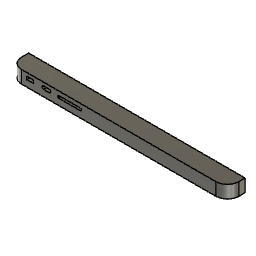
laptop side reference model v4 (Autodesk Fusion 360 design; units mm, degrees)
Autodesk Fusion 360 part; units mm, degrees
sketch "Sketch1" plane through (0, 0, 0) normal (0, 0, 1) x (1, 0, 0) in component "Laptop side"
  line L0 (0, 0) -> (225.9, 0)
  line L1 (225.9, 0) -> (225.9, 18.5)
  line L2 (225.9, 18.5) -> (0, 18.5)
  line L3 (0, 18.5) -> (0, 0)
  dimension "d1" = 225.9
  dimension "d2" = 18.5
  constraint horizontal L0
  constraint vertical L1
  constraint horizontal L2
  constraint vertical L3
  constraint coincident L0.start L3.end
  measures "d1" distance of L0.start L0.end
  measures "d2" distance of L0.end L1.end
extrude "Extrude1" add sketch "Sketch1" along normal blind 13.24 in component "Laptop side"
sketch "Sketch2" plane through (0, 0, 0) normal (0, -1, 0) x (1, 0, 0) in component "Laptop side"
  line L0 (0, 0) -> (225.9, 0)
  line L1 (225.9, 0) -> (225.9, 13.24)
  line L2 (225.9, 13.24) -> (0, 13.24)
  line L3 (0, 13.24) -> (0, 0)
  line L4 (16.56, 9.86) -> (23.66, 9.86)
  line L5 (23.66, 9.86) -> (23.66, 6.76)
  line L6 (23.66, 6.76) -> (16.56, 6.76)
  line L7 (16.56, 6.76) -> (16.56, 9.86)
  line L8 (33.96, 9.82) -> (40.16, 9.82)
  line L9 (41.56, 8.42) -> (41.56, 8.04)
  line L10 (40.16, 6.64) -> (33.96, 6.64)
  line L11 (32.56, 8.04) -> (32.56, 8.42)
  arc A0 (33.96, 9.82) -> (32.56, 8.42) centre (33.96, 8.42) ccw
  arc A1 (32.56, 8.04) -> (33.96, 6.64) centre (33.96, 8.04) ccw
  arc A2 (40.16, 6.64) -> (41.56, 8.04) centre (40.16, 8.04) ccw
  arc A3 (41.56, 8.42) -> (40.16, 9.82) centre (40.16, 8.42) ccw
  line L12 (49.66, 9.04) -> (72.76, 9.04)
  line L13 (73.46, 8.34) -> (73.46, 7.34)
  line L14 (72.76, 6.64) -> (49.66, 6.64)
  line L15 (48.96, 7.34) -> (48.96, 8.34)
  arc A4 (49.66, 9.04) -> (48.96, 8.34) centre (49.66, 8.34) ccw
  arc A5 (48.96, 7.34) -> (49.66, 6.64) centre (49.66, 7.34) ccw
  arc A6 (72.76, 6.64) -> (73.46, 7.34) centre (72.76, 7.34) ccw
  arc A7 (73.46, 8.34) -> (72.76, 9.04) centre (72.76, 8.34) ccw
  point P0 (32.56, 9.82)
  point P1 (41.56, 9.82)
  point P2 (32.56, 6.64)
  point P3 (48.96, 9.04)
  point P4 (73.46, 9.04)
  point P5 (48.96, 6.64)
  dimension "d5" = 7.1
  dimension "d6" = 3.1
  dimension "d7" = 16.56
  dimension "d8" = 3.38
  dimension "d19" = 9
  dimension "d20" = 3.18
  dimension "d21" = 1.4
  dimension "d22" = 3.42
  dimension "d24" = 25
  dimension "d25" = 8.9
  dimension "d26" = 24.5
  dimension "d27" = 2.4
  dimension "d28" = 4.2
  dimension "d29" = 56.9
  dimension "d30" = 25.3
  dimension "d31" = 0.7
  constraint horizontal L4
  constraint vertical L5
  constraint horizontal L6
  constraint vertical L7
  constraint horizontal L8
  constraint vertical L9
  constraint horizontal L10
  constraint vertical L11
  constraint coincident P0 L8
  constraint coincident P0 L11
  constraint tangent L8 A0
  constraint tangent L11 A0
  constraint coincident P2 L10
  constraint coincident P2 L11
  constraint tangent L10 A1
  constraint tangent L11 A1
  constraint equal A0 A1
  constraint tangent L9 A2
  constraint tangent L10 A2
  constraint equal A0 A2
  constraint coincident P1 L8
  constraint coincident P1 L9
  constraint tangent L8 A3
  constraint tangent L9 A3
  constraint equal A0 A3
  constraint horizontal L12
  constraint vertical L13
  constraint horizontal L14
  constraint vertical L15
  constraint coincident P3 L12
  constraint coincident P3 L15
  constraint tangent L12 A4
  constraint tangent L15 A4
  constraint coincident P5 L14
  constraint coincident P5 L15
  constraint tangent L14 A5
  constraint tangent L15 A5
  constraint equal A4 A5
  constraint tangent L13 A6
  constraint tangent L14 A6
  constraint equal A4 A6
  constraint coincident P4 L12
  constraint coincident P4 L13
  constraint tangent L12 A7
  constraint tangent L13 A7
  constraint equal A4 A7
  measures "d5" distance of L4.start L4.end
  measures "d6" distance of L4.start L6.end
  measures "d7" distance of L3 L7
  measures "d8" distance of L2 L4
  measures "d19" distance of P0 P1
  measures "d20" distance of P0 P2
  measures "d21" radius of A0
  measures "d22" distance of L2 L8
  measures "d24" distance of L7 L9
  measures "d25" distance of L5 L11
  measures "d26" distance of P3 P4
  measures "d27" distance of P3 P5
  measures "d28" distance of L2 L12
  measures "d29" distance of L7 L13
  measures "d30" distance of L5 L15
  measures "d31" radius of A4
extrude "Extrude2" cut sketch "Sketch2" against normal blind 9.5 contours L4 L5 L6 L7 | L8 L9 L10 L11 A0 A1 A2 A3 | L12 L13 L14 L15 A4 A5 A6 A7 in component "Laptop side"
fillet "Fillet1" radius 12 1 edges at (225.9, 0, 6.62) in component "Laptop side"
fillet "Fillet1" radius 11 1 edges at (0, 0, 6.62) in component "Laptop side"
component "Laptop side" placed x (1, 0, 0) y (0, 1, 0) z (0, 0, 1) at (0, 0, 0)
